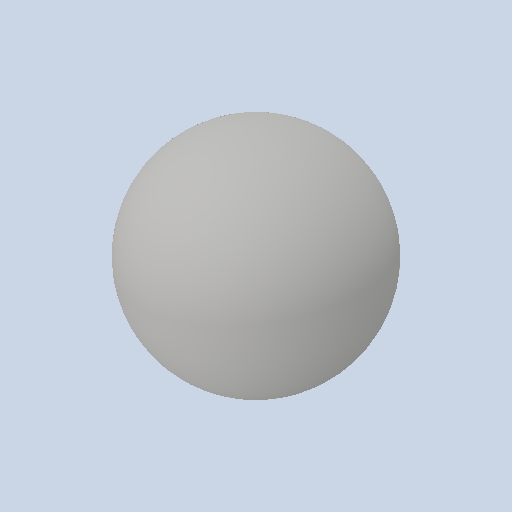
# Autodesk Inventor part: 040400DR-22-H4W(0_5)3_ball_CPY
Saved by Autodesk Inventor 2024 (Build 280153000, 153)
## iProperties
Created: 2023-06-17
Part Number: 040400DR-22-H4W(0_5)3_ball_CPY
Material: Generic
Catalog Web Link: www.cadenas.de
Description: DR-H ball-D-Series bearings
Vendor: TOKBEARING
Document SubType Name: Modeling
Designer: zegi
Manufacturer: TOKBEARING
Mass: 8300 g
Surface Area: 0.448883 cm^2
Volume: 0.0282796 cm^3
Density: 1 g/cm^3
Appearance: PSOLRGB-175-175-175
Category: PARTsolutions
Company: TOKBEARING
Title: 040400DR-22-H4W(0.5)3_ball
Author: Cadenas PARTsolutions
Comments: D-Series bearings
PSOL_IDENT_0: {$CADENAS_DATA/23d-libs/tok_bearing/d_series_bearings/dr_h/dr_h_ball.prj},197 {VTYP=3D},{NB=040400DR
PSOL_IDENT_1: -22-H4W(0.5)3_ball},{LINA=040400DR-22-H4W(0.5)3_ball},{NN=DR-H ball},{DATE=16.12.2020 00:38:04},{GEO
PSOL_IDENT_2: MDATE=19.02.2013 00:00:00},{VERSION=},{LINEID=1750},{WBVAR=},{WBNUMERIC=}  {NB=040400DR-22-H4W(0.5)3
PSOL_IDENT_3: _ball},{LINA=040400DR-22-H4W(0.5)3_ball},{KT=DUMMY},{IDNR=},{CODE=040400},{PN=DR-22-H4W(0.5)3},{D=22
PSOL_IDENT_4: },{SD=4.0},{W=7.0},{W1=0.5},{W1X=0.500},{W2=3},{W2X=3.000},{LOAD=196 (20)},{TYPE=12},{QTY=1.000},{GW=
PSOL_IDENT_5: 8.3},{BD=3.78},{OP=40.2862},{N=5},{R=6.415},{GP=3.64}
NB: 040400DR-22-H4W(0.5)3_ball
NN: DR-H ball
NT: D-Series bearings
NBSYN: $CODE.$PN._ball
LINA: 040400DR-22-H4W(0.5)3_ball
CATALOG: TOK, Inc
CODE: 040400
PN: DR-22-H4W(0.5)3
D: 22
SD: 4
W: 7
W1: 0.5
W2: 3
LOAD: 196 (20)
TYPE: 12
QTY: 1.000
GW: 8.3
SUPPLIER: TOKBEARING
ARTICLENO: 040400DR-22-H4W(0.5)3_ball
BOMINFO: 040400DR-22-H4W(0.5)3_ball
CREATOR: CADENAS GmbH
Autodesk Inventor part; units mm, degrees
sketch "Sketch_1" plane through (0, 0, 0) normal (0, 0, 1) x (1, 0, 0)
  line L0 (1.89, 0) -> (-1.89, 0)
  arc A0 (1.89, 0) -> (-1.89, 0) centre (0, 0) ccw
  line L1 (1.89, 0) -> (-1.89, 0)
  constraints: 4 end point, 2 point on circle, 1 centre point
revolve "Revolution1" add sketch "Sketch_1" angle 360 about axis through (1.89, 0, 0) along (1, 0, 0)
ref_plane "Ball_OR_XY" through (0, 0, 0) normal (1, 0, 0) x (0, 0, -1)
ref_plane "Ball_OR_YZ" through (0, 0, 0) normal (0, 0, -1) x (0, 1, 0)
ref_plane "Ball_OR_ZX" through (0, 0, 0) normal (0, 1, 0) x (1, 0, 0)
body "Solid1"
